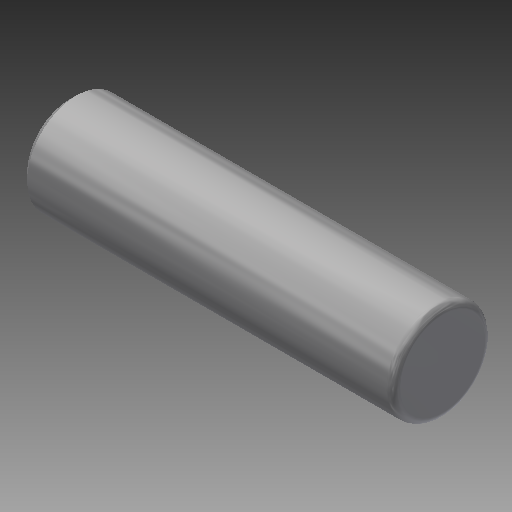
# Autodesk Inventor part: Shaft
Saved by Autodesk Inventor 2017 (Build 210142000, 142)
## iProperties
Created: 2016-12-06
Part Number: Shaft
Material: Steel
Document SubType Name: Modeling
Designer: aesen
Density: 1 g/cm^3
Appearance: Steel
CustomPartVersion: 1
Author: aesen
Autodesk Inventor part; units mm, degrees
ref_plane "Start Plane" through (0, 0, 0) normal (1, 0, 0) x (0, 1, 0)
ref_plane "XZ Plane" through (0, 0, 0) normal (0, 1, 0) x (-1, 0, 0)
ref_plane "XY Plane" through (0, 0, 0) normal (0, 0, 1) x (1, 0, 0)
sketch "Main Sketch" plane through (0, 0, 0) normal (0, 0, 1) x (1, 0, 0)
  line L0 (0, 0) -> (132.08, 0)
  line L1 (0, 0) -> (0, 17.4625)
  line L2 (132.08, 17.4625) -> (132.08, 0)
  line L3 (0, 17.4625) -> (132.08, 17.4625)
  dimension "d3" = 34.925
  constraints: 8 end point, 3 horizontal, 2 vertical
  measures "d3" diameter of L3 L0
revolve "Revolution1" add sketch "Main Sketch" angle 360 about axis through (0, 0, 0) along (1, 0, 0)
chamfer "Chamfer1" distance 2.54 angle 45 1 edges at (0, -17.4625, 0) measured on face at (88.0533, 17.4059, -1.4051)
fillet "Fillet1" radius 2.54 1 edges at (132.08, -17.4625, 0)
body "Solid1"
